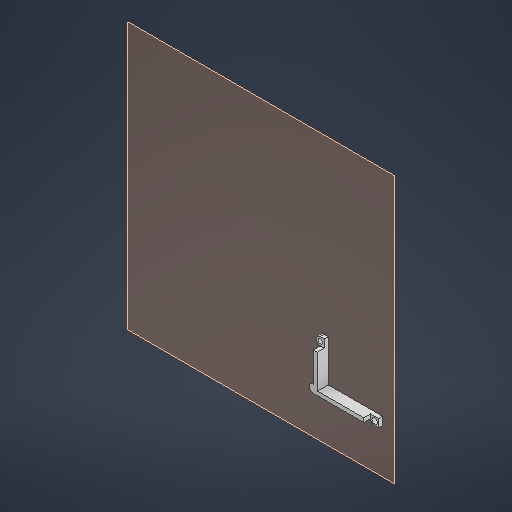
# Autodesk Inventor part: rightbmw
Saved by Autodesk Inventor 2026.2 (Build 302298010, 298A)
## iProperties
Created: 2026-09-07
Part Number: rightbmw
Material: Generic
Document SubType Name: Modeling
Designer: karol
Density: 1 g/cm^3
Appearance: Default
Author: karol
Autodesk Inventor part; units mm, degrees
ref_plane "YZ Plane" through (0, 0, 0) normal (1, 0, 0) x (0, 1, 0)
ref_plane "XZ Plane" through (0, 0, 0) normal (0, 1, 0) x (-1, 0, 0)
ref_plane "XY Plane" through (0, 0, 0) normal (0, 0, 1) x (1, 0, 0)
sketch "Sketch1" plane through (0, 0, 0) normal (0, 0, 1) x (1, 0, 0)
  line L0 (90, -35) -> (46.6, -35) projected
  line L1 (90, -35) -> (90, 35) projected
  line L2 (90, 35) -> (46.6, 35) projected
  line L3 (49.6, 32) -> (87, 32) projected
  line L4 (87, 32) -> (87, -32) projected
  line L5 (87, -32) -> (49.6, -32) projected
  line L6 (-58, -60) -> (-60, -60) projected
  line L7 (-60, -60) -> (-60, -39.5) projected
  line L8 (-60, -39.5) -> (-58, -39.5) projected
  line L9 (-58, -39.5) -> (-58, -60) projected
  line L10 (49.6, 30) -> (51.6, 30) projected
  line L11 (51.6, 30) -> (51.6, 9.5) projected
  line L12 (51.6, 9.5) -> (49.6, 9.5) projected
  line L13 (49.6, 9.5) -> (49.6, 30) projected
  line L14 (-58, 39.5) -> (-60, 39.5) projected
  line L15 (-60, 39.5) -> (-60, 60) projected
  line L16 (-60, 60) -> (-58, 60) projected
  line L17 (-58, 60) -> (-58, 39.5) projected
  line L18 (-21.6, -39.5) -> (-19.6, -39.5) projected
  line L19 (-19.6, -39.5) -> (-19.6, -60) projected
  line L20 (-19.6, -60) -> (-21.6, -60) projected
  line L21 (-21.6, -60) -> (-21.6, -39.5) projected
  line L22 (51.6, -30) -> (49.6, -30) projected
  line L23 (49.6, -30) -> (49.6, -9.5) projected
  line L24 (49.6, -9.5) -> (51.6, -9.5) projected
  line L25 (51.6, -9.5) -> (51.6, -30) projected
  line L26 (-21.6, 60) -> (-19.6, 60) projected
  line L27 (-19.6, 60) -> (-19.6, 39.5) projected
  line L28 (-19.6, 39.5) -> (-21.6, 39.5) projected
  line L29 (-21.6, 39.5) -> (-21.6, 60) projected
  line L30 (90, -35) -> (90, 35) projected
  line L31 (90, 35) -> (49.6, 35) projected
  line L32 (49.6, 35) -> (49.6, 60) projected
  line L33 (49.6, 60) -> (90, 60) projected
  line L34 (90, 60) -> (90, 90) projected
  line L35 (90, 90) -> (-19.6, 90) projected
  line L36 (-19.6, 90) -> (-19.6, 65) projected
  line L37 (-19.6, 65) -> (-60, 65) projected
  line L38 (-60, 65) -> (-60, 90) projected
  line L39 (-60, 90) -> (-90, 90) projected
  line L40 (-90, 90) -> (-90, -90) projected
  line L41 (-90, -90) -> (-60, -90) projected
  line L42 (-60, -90) -> (-60, -65) projected
  line L43 (-60, -65) -> (-19.6, -65) projected
  line L44 (-19.6, -65) -> (-19.6, -90) projected
  line L45 (-19.6, -90) -> (90, -90) projected
  line L46 (90, -90) -> (90, -60) projected
  line L47 (90, -60) -> (49.6, -60) projected
  line L48 (49.6, -60) -> (49.6, -35) projected
  line L49 (49.6, -35) -> (90, -35) projected
  line L50 (86, -32) -> (73.8, -32) projected
  line L51 (73.8, -32) -> (73.8, -7.5) projected
  line L52 (73.8, -7.5) -> (86, -7.5) projected
  line L53 (86, -7.5) -> (86, -32) projected
  line L54 (65.8, -32) -> (53.6, -32) projected
  line L55 (53.6, -32) -> (53.6, -7.5) projected
  line L56 (53.6, -7.5) -> (65.8, -7.5) projected
  line L57 (65.8, -7.5) -> (65.8, -32) projected
  line L58 (86, -86) -> (70.6, -86) projected
  line L59 (70.6, -86) -> (70.6, -69.8) projected
  line L60 (70.6, -69.8) -> (86, -69.8) projected
  line L61 (86, -69.8) -> (86, -86) projected
  line L62 (86, 86) -> (86, 69.8) projected
  line L63 (86, 69.8) -> (70.6, 69.8) projected
  line L64 (70.6, 69.8) -> (70.6, 86) projected
  line L65 (70.6, 86) -> (86, 86) projected
  line L66 (73.8, 32) -> (86, 32) projected
  line L67 (86, 32) -> (86, 7.5) projected
  line L68 (86, 7.5) -> (73.8, 7.5) projected
  line L69 (73.8, 7.5) -> (73.8, 32) projected
  line L70 (65.8, 32) -> (65.8, 7.5) projected
  line L71 (65.8, 7.5) -> (53.6, 7.5) projected
  line L72 (53.6, 7.5) -> (53.6, 32) projected
  line L73 (53.6, 32) -> (65.8, 32) projected
  line L74 (-69.6, -87) -> (-85, -87) projected
  line L75 (-85, -87) -> (-85, -70.8) projected
  line L76 (-85, -70.8) -> (-69.6, -70.8) projected
  line L77 (-69.6, -70.8) -> (-69.6, -87) projected
  line L78 (-56, -62) -> (-56, -37.5) projected
  line L79 (-56, -37.5) -> (-43.8, -37.5) projected
  line L80 (-43.8, -37.5) -> (-43.8, -62) projected
  line L81 (-43.8, -62) -> (-56, -62) projected
  line L82 (-56, 62) -> (-43.8, 62) projected
  line L83 (-43.8, 62) -> (-43.8, 37.5) projected
  line L84 (-43.8, 37.5) -> (-56, 37.5) projected
  line L85 (-56, 37.5) -> (-56, 62) projected
  line L86 (-23.6, 62) -> (-23.6, 37.5) projected
  line L87 (-23.6, 37.5) -> (-35.8, 37.5) projected
  line L88 (-35.8, 37.5) -> (-35.8, 62) projected
  line L89 (-35.8, 62) -> (-23.6, 62) projected
  line L90 (-23.6, -62) -> (-35.8, -62) projected
  line L91 (-35.8, -62) -> (-35.8, -37.5) projected
  line L92 (-35.8, -37.5) -> (-23.6, -37.5) projected
  line L93 (-23.6, -37.5) -> (-23.6, -62) projected
  line L94 (-85, 87) -> (-69.6, 87) projected
  line L95 (-69.6, 87) -> (-69.6, 70.8) projected
  line L96 (-69.6, 70.8) -> (-85, 70.8) projected
  line L97 (-85, 70.8) -> (-85, 87) projected
  line L98 (49.6, -35) -> (46.6, -35)
  line L99 (46.6, -35) -> (46.6, -60)
  line L100 (46.6, -60) -> (49.6, -60)
  line L101 (49.6, -60) -> (49.6, -35)
  line L102 (46.6, -60) -> (90, -60)
  line L103 (90, -60) -> (90, -63)
  line L104 (90, -63) -> (46.6, -63)
  line L105 (46.6, -63) -> (46.6, -60)
  circle A0 centre (-63, -65) radius 1.5 projected
  circle A1 centre (-16.6, -87) radius 1.5 projected
  circle A2 centre (49.6, -87) radius 1.5 projected
  circle A3 centre (46.6, -60) radius 1.5 projected
  circle A4 centre (87, -63) radius 1.5 projected
  circle A5 centre (46.6, -32) radius 1.5 projected
  circle A6 centre (46.6, 32) radius 1.5 projected
  circle A7 centre (87, 63) radius 1.5 projected
  circle A8 centre (46.6, 60) radius 1.5 projected
  circle A9 centre (49.6, 87) radius 1.5 projected
  circle A10 centre (-16.6, 87) radius 1.5 projected
  circle A11 centre (-16.6, 65) radius 1.5 projected
  circle A12 centre (-63, 65) radius 1.5 projected
  line L106 (-76, -39.25) -> (-82, -39.25) projected
  line L107 (-82, -39.25) -> (-82, -20.75) projected
  line L108 (-82, -20.75) -> (-76, -20.75) projected
  line L109 (-76, -20.75) -> (-76, -39.25) projected
  line L110 (-76, 20.75) -> (-82, 20.75) projected
  line L111 (-82, 20.75) -> (-82, 39.25) projected
  line L112 (-82, 39.25) -> (-76, 39.25) projected
  line L113 (-76, 39.25) -> (-76, 20.75) projected
  circle A13 centre (-86.5, -55.7158) radius 1.25 projected
  circle A14 centre (-86.5, 55.8) radius 1.25 projected
  circle A15 centre (-79.5, -5.4579) radius 1.25 projected
  circle A16 centre (-79.5, 5.5421) radius 1.25 projected
  arc A17 (46.6, 35) -> (49.6, 32) centre (46.6, 32) ccw projected
  arc A18 (49.6, -32) -> (46.6, -35) centre (46.6, -32) ccw projected
  point P0 (0, 0)
  point P1 (49.6, 29)
  point P2 (49.6, -29)
  dimension "d0" = 3
  dimension "d1" = 25
  dimension "d2" = 3
  constraints: 16 end point, 4 parallel, 2 horizontal, 2 perpendicular, 1 point on line
  measures "d0" distance of L100.end L99.end
  measures "d1" distance of L99.end L98.end
  measures "d2" distance of L102.end L103.end
extrude "Extrusion1" add sketch "Sketch1" along normal blind 8 contours L48 L100 A3 L99 L0 | L47 L46 L104 A4 L105 A3 L100 | A3 L100 L99 | A3 L105 L100 | L104 A4 picked at (87.0603, -62.5036)
ref_plane "Work Plane1" through (0, 0, 0) normal (0, 0, 1) x (1, 0, 0)
sketch "Sketch2" plane through (0, 0, 0) normal (0, 0, 1) x (1, 0, 0)
  line L0 (90, -35) -> (46.6, -35) projected
  line L1 (90, -35) -> (90, 35) projected
  line L2 (90, 35) -> (46.6, 35) projected
  line L3 (49.6, 32) -> (87, 32) projected
  line L4 (87, 32) -> (87, -32) projected
  line L5 (87, -32) -> (49.6, -32) projected
  line L6 (49.6, -60) -> (49.6, -35) projected
  line L7 (43.6, -29) -> (49.6, -29)
  line L8 (49.6, -29) -> (49.6, -35)
  line L9 (49.6, -35) -> (43.6, -35)
  line L10 (43.6, -35) -> (43.6, -29)
  arc A0 (46.6, 35) -> (49.6, 32) centre (46.6, 32) ccw projected
  arc A1 (49.6, -32) -> (46.6, -35) centre (46.6, -32) ccw projected
  point P0 (0, 0)
  point P1 (43.6, -32)
  point P2 (46.6, -35)
  point P3 (46.6, -29)
  point P4 (49.6, -32)
  point P5 (49.6, -32)
  constraints: 8 end point, 2 parallel, 1 horizontal, 1 perpendicular
extrude "Extrusion2" add sketch "Sketch2" along normal blind 3 contours L0 L8 L5 L4 L3 A0 L2 L1 | L0 A1 L8 | A1 L7 L8
sketch "Sketch3" plane through (0, 0, 0) normal (0, 0, -1) x (-1, 0, 0)
  line L0 (-49.6, -29) -> (-43.6, -29) projected
  line L1 (-49.6, -35) -> (-49.6, -29) projected
  line L2 (-43.6, -29) -> (-49.6, -29)
  line L3 (-49.6, -29) -> (-49.6, -35)
  line L4 (-49.6, -35) -> (-43.6, -35)
  line L5 (-43.6, -35) -> (-43.6, -29)
  line L6 (-49.6, -29) -> (-43.6, -35)
  line L7 (-49.6, -35) -> (-43.6, -29)
  circle A0 centre (-46.6, -32) radius 1.65
  point P0 (0, 0)
  dimension "d7" = 3.3
  constraints: 12 end point, 2 parallel, 2 perpendicular, 1 centre point, 1 horizontal, 1 midpoint
  measures "d7" diameter of A0
extrude "Extrusion3" cut sketch "Sketch3" against normal blind 3 contours A0 L7 L6 | L6 L7 A0 | A0 L6 L7 | L7 L6 A0
sketch "Sketch4" plane through (46.6, -63, 0) normal (0, -1, 0) x (1, 0, 0)
  line L0 (0, 8) -> (43.4, 8) projected
  line L1 (43.4, 8) -> (37.4, 8)
  line L2 (37.4, 8) -> (37.4, 3)
  line L3 (37.4, 3) -> (43.4, 3)
  line L4 (43.4, 3) -> (43.4, 8)
  line L5 (37.4, 3) -> (43.4, 3)
  line L6 (43.4, 3) -> (43.4, 0)
  line L7 (43.4, 0) -> (37.4, 0)
  line L8 (37.4, 0) -> (37.4, 3)
  point P0 (-46.6, 0)
  dimension "d10" = 6
  dimension "d11" = 5
  constraints: 16 end point, 4 parallel, 2 horizontal, 2 perpendicular, 1 point on line
  measures "d10" distance of L3.end L2.end
  measures "d11" distance of L2.end L1.end
extrude "Extrusion4" cut sketch "Sketch4" against normal blind 3 contours L0 L4 L3 L2
extrude "Extrusion5" add sketch "Sketch4" along normal blind 3 contours L3 L6 L7 L8
sketch "Sketch5" plane through (84, -60, 3) normal (0, 0, 1) x (1, 0, 0)
  line L0 (0, 0) -> (6, 0) projected
  line L1 (6, 0) -> (6, -6) projected
  line L2 (0, 0) -> (6, -6)
  line L3 (6, -6) -> (0, -6)
  line L4 (0, -6) -> (6, 0)
  circle A0 centre (3, -3) radius 2
  point P0 (-84, 60)
  dimension "d16" = 4
  constraints: 6 end point, 2 perpendicular, 1 centre point, 1 midpoint
  measures "d16" diameter of A0
extrude "Extrusion6" cut sketch "Sketch5" against normal blind 3 contours A0 L4 L2 | L2 L4 A0 | A0 L2 L4 | L2 A0 L4
sketch "Sketch6" plane through (0, 0, 8) normal (0, 0, 1) x (1, 0, 0)
  line L0 (90, -60) -> (49.6, -60) projected
  line L1 (46.6, -63) -> (84, -63) projected
  line L2 (49.6, -63) -> (43.6, -63)
  line L3 (43.6, -63) -> (43.6, -57)
  line L4 (43.6, -57) -> (49.6, -57)
  line L5 (49.6, -57) -> (49.6, -63)
  point P0 (0, 0)
  dimension "d23" = 6
  dimension "d24" = 6
  constraints: 8 end point, 2 parallel, 1 horizontal, 1 perpendicular, 1 point on line
  measures "d23" distance of L3.end L4.end
  measures "d24" distance of L2.end L3.end
extrude "Extrusion8" add sketch "Sketch6" against normal blind 8
sketch "Sketch7" plane through (0, 0, 0) normal (0, 0, -1) x (-1, 0, 0)
  circle A0 centre (-46.6, -60) radius 2
  line L0 (-43.6, -57) -> (-46.6, -57) projected
  line L1 (-43.6, -63) -> (-84, -63) projected
  line L2 (-43.6, -57) -> (-43.6, -63)
  line L3 (-43.6, -63) -> (-49.6, -57)
  line L4 (-49.6, -60) -> (-49.6, -35) projected
  line L5 (-43.6, -57) -> (-49.6, -57)
  line L6 (-49.6, -63) -> (-49.6, -57)
  line L7 (-49.6, -63) -> (-43.6, -57)
  circle A1 centre (-46.6, -60) radius 1.65
  point P0 (0, 0)
  point P1 (-49.6, -29)
  dimension "d27" = 4
  dimension "d28" = 3.3
  constraints: 10 end point, 4 perpendicular, 2 centre point, 2 coincident, 1 midpoint, 1 point on line
  measures "d27" diameter of A0
  measures "d28" diameter of A1
extrude "Extrusion9" cut sketch "Sketch7" against normal blind 6 contours A0 L3 A1 L7 | L7 A1 L3 A0 | A0 L7 A1 L3 | L3 A1 L7 A0 | A1 L3 L7 | L7 L3 A1 | A1 L7 L3 | L3 L7 A1
fillet "Fillet1" radius 3 2 edges at (43.6, -57, 4) (43.6, -63, 4)
fillet "Fillet2" radius 3 1 edges at (84, -66, 1.5)
sketch "Sketch8" plane through (0, 0, 3) normal (0, 0, 1) x (1, 0, 0)
  line L0 (49.6, -35) -> (90, -35) projected
  line L1 (90, -35) -> (90, 35) projected
  line L2 (49.6, -35) -> (90, -35)
  line L3 (90, -35) -> (90, 35)
  line L4 (90, 35) -> (49.6, 35)
  line L5 (49.6, 35) -> (49.6, -35)
  line L6 (49.6, 35) -> (43.6, 35)
  line L7 (43.6, 35) -> (43.6, 29)
  line L8 (43.6, 29) -> (49.6, 29)
  line L9 (49.6, 29) -> (49.6, 35)
  circle A0 centre (46.6, -32) radius 1.65 projected
  line L10 (49.6, -29) -> (46.6, -29) projected
  arc A1 (46.6, -29) -> (46.6, -35) centre (46.6, -32) ccw projected
  line L11 (49.6, -35) -> (46.6, -35) projected
  line L12 (49.6, -35) -> (90, -35) projected
  line L13 (90, -35) -> (90, 35) projected
  line L14 (90, 35) -> (46.6, 35) projected
  arc A2 (46.6, 35) -> (49.6, 32) centre (46.6, 32) ccw projected
  line L15 (49.6, 32) -> (87, 32) projected
  line L16 (87, 32) -> (87, -32) projected
  line L17 (87, -32) -> (49.6, -32) projected
  line L18 (49.6, -32) -> (49.6, -29) projected
  circle A3 centre (46.6, 32) radius 3
  point P0 (0, 0)
  point P1 (46.6, 35)
  dimension "d33" = 6
  dimension "d34" = 6
  constraints: 16 end point, 4 parallel, 2 horizontal, 2 perpendicular, 1 coincident, 1 midpoint, 1 vertical alignment, 2 other
  measures "d33" distance between parallel lines of L5 L7
  measures "d34" distance from line of point (46.6, 35) L8
extrude "Extrusion10" cut sketch "Sketch8" against normal blind 3 contours L5 L17 L16 L15 L4 L1 L0 | L5 A3 L6 | A2 A3
body "Solid1"
